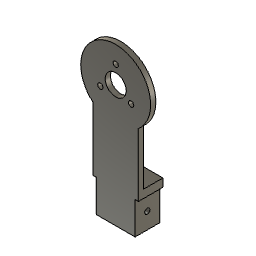
Upper structure (Autodesk Fusion 360 design; units mm, degrees)
Autodesk Fusion 360 part; units mm, degrees
sketch "Esquisse1" plane through (0, 0, 0) normal (0, 1, 0) x (1, 0, 0)
  circle A0 centre (0, -25) radius 21.6
  line L0 (0, 15.5) -> (14, 15.5)
  line L1 (0, 15.5) -> (-14, 15.5)
  line L2 (-14, 15.5) -> (-14, -8.5513)
  line L3 (14, 15.5) -> (14, -8.5513)
  circle A1 centre (0, -25) radius 6
  circle A2 centre (0, -36) radius 1.625
  circle A3 centre (-9.5263, -19.5) radius 1.625
  circle A4 centre (9.5263, -19.5) radius 1.625
  dimension "d1" = 43.2
  dimension "d4" = 14
  dimension "d5" = 14
  dimension "d9" = 11
  dimension "d12" = 12
  dimension "d64" = 3.25
  dimension "d65" = 3.25
  dimension "d66" = 3.25
  constraint coincident A0 L2.end
  constraint perpendicular L1 L2
  constraint coincident A0 L3.end
  constraint perpendicular L0 L3
  measures "d1" diameter of A0
  measures "d4" distance of L0.start L0.end
  measures "d5" distance of L0.start L1.end
  measures "d9" distance of A0.centre A4.centre
  measures "d12" diameter of A1
  measures "d64" diameter of A2
  measures "d65" diameter of A3
  measures "d66" diameter of A4
extrude "Extrusion1" add sketch "Esquisse1" along normal blind 3.2 contours A0 | A2 | A3 | A4
extrude "Extrusion2" add sketch "Esquisse1" along normal blind 3.2 contours A0 L0 L1 L2 L3
sketch "Esquisse2" plane through (0, 0, -15.5) normal (0, 0, -1) x (1, 0, 0)
  line L0 (14, 0) -> (-14, 0)
  line L1 (-14, 0) -> (-14, -3.2)
  line L2 (-14, -3.2) -> (14, -3.2)
  line L3 (14, -3.2) -> (14, 0)
  line L4 (-14, -3.2) -> (14, -3.2)
  dimension "d17" = 28
  constraint horizontal L4
  constraint coincident L1.end L2.start
  measures "d17" distance of L1.end L2.end
extrude "Extrusion3" add sketch "Esquisse2" along normal blind 10
sketch "Esquisse3" plane through (0, 0, -25.5) normal (0, 0, -1) x (1, 0, 0)
  line L0 (-14, 0) -> (-14, -3.2)
  line L1 (-14, -3.2) -> (14, -3.2)
  line L2 (14, -3.2) -> (14, 0)
  line L3 (14, 0) -> (-14, 0)
extrude "Extrusion4" cut sketch "Esquisse3" against normal blind 10
extrude "Extrusion5" add sketch "Esquisse2" along normal blind 5
sketch "Esquisse4" plane through (0, 0, -20.5) normal (0, 0, -1) x (1, 0, 0)
  line L0 (-14, -3.2) -> (14, -3.2)
  line L1 (14, -3.2) -> (14, 0)
  line L2 (14, 0) -> (-14, 0)
  line L3 (-14, 0) -> (-14, -3.2)
  line L4 (-14, -3.2) -> (-14, -15.2)
  line L5 (-14, -15.2) -> (14, -15.2)
  line L6 (14, -15.2) -> (14, -3.2)
  dimension "d25" = 12
  constraint vertical L4
  constraint horizontal L5
  constraint vertical L6
  constraint coincident L0.end L1.start
  measures "d25" distance of L0.end L5.end
extrude "Extrusion6" add sketch "Esquisse4" along normal blind 10
sketch "Esquisse5" plane through (0, 0, -20.5) normal (0, 0, 1) x (-1, 0, 0)
  line L0 (14, -3.2) -> (-14, -3.2)
  line L1 (-14, -3.2) -> (-14, -15.2)
  line L2 (-14, -15.2) -> (14, -15.2)
  line L3 (14, -15.2) -> (14, -3.2)
  line L4 (-14, -3.2) -> (-7.5, -3.2)
  line L5 (14, -3.2) -> (7.5, -3.2)
  line L6 (-7.5, -3.2) -> (-7.5, -6.7)
  line L7 (7.5, -3.2) -> (7.5, -6.7)
  circle A0 centre (-7.5, -6.7) radius 1.625
  circle A1 centre (7.5, -6.7) radius 1.625
  dimension "d28" = 6.5
  dimension "d29" = 6.5
  dimension "d32" = 3.5
  dimension "d33" = 3.5
  dimension "d34" = 3.25
  dimension "d35" = 3.25
  constraint coincident L0.end L1.start
  constraint perpendicular L1 L4
  constraint coincident L0.start L3.end
  constraint perpendicular L3 L5
  constraint perpendicular L0 L6
  constraint perpendicular L0 L7
  constraint coincident L6.end A0.centre
  constraint coincident L7.end A1.centre
  measures "d28" distance of L0.end L4.end
  measures "d29" distance of L0.start L5.end
  measures "d32" distance of L4.end L6.end
  measures "d33" distance of L5.end L7.end
  measures "d34" diameter of A0
  measures "d35" diameter of A1
extrude "Extrusion7" cut sketch "Esquisse5" against normal blind 8 contours A0
extrude "Extrusion8" cut sketch "Esquisse5" against normal blind 8 contours A1
sketch "Esquisse6" plane through (0, 0, -20.5) normal (0, 0, 1) x (-1, 0, 0)
  circle A0 centre (7.5, -6.7) radius 1.625
  circle A1 centre (-7.5, -6.7) radius 1.625
  line L0 (14, -3.2) -> (-14, -3.2)
  line L1 (-14, -3.2) -> (-14, -15.2)
  line L2 (-14, -15.2) -> (14, -15.2)
  line L3 (14, -15.2) -> (14, -3.2)
  line L4 (0, -3.2) -> (0, -10.7)
  dimension "d40" = 7.5
  constraint midpoint L0 L4.start
  constraint perpendicular L0 L4
  measures "d40" distance of L4.start L4.end
sketch "Esquisse7" plane through (0, 0, -30.5) normal (0, 0, -1) x (1, 0, 0)
  line L0 (14, -15.2) -> (14, 0)
  line L1 (14, 0) -> (-14, 0)
  line L2 (-14, 0) -> (-14, -15.2)
  line L3 (-14, -15.2) -> (14, -15.2)
  circle A0 centre (0, -7.6) radius 6.4
  circle A1 centre (0, -7.6) radius 3.865
  dimension "d56" = 7.73
  constraint concentric A0 A1
  measures "d56" diameter of A1
extrude "Extrusion9" add sketch "Esquisse7" along normal blind 20 contours A0 | A1
sketch "Esquisse8" plane through (0, 0, 0) normal (1, 0, 0) x (0, 1, 0)
sketch "Esquisse9" plane through (0, 0, 0) normal (0, 0, 1) x (1, 0, 0)
sketch "Esquisse10" plane through (0, 0, 0) normal (0, 0, 1) x (1, 0, 0)
sketch "Esquisse11" plane through (0, 0, 0) normal (1, 0, 0) x (0, 1, 0)
sketch "Esquisse12" plane through (-14, 0, 0) normal (-1, 0, 0) x (0, -1, 0)
  line L0 (0, -30.5) -> (0, 8.5513)
  line L1 (0, 8.5513) -> (-3.2, 8.5513)
  line L2 (-3.2, 8.5513) -> (-3.2, -20.5)
  line L3 (-3.2, -20.5) -> (-15.2, -20.5)
  line L4 (-15.2, -20.5) -> (-15.2, -30.5)
  line L5 (-15.2, -30.5) -> (0, -30.5)
  line L6 (-15.2, -25.5) -> (-7.6, -25.5)
  line L7 (-7.6, -25.5) -> (-7.6, -40.5)
  circle A0 centre (-7.6, -40.5) radius 1.625
  dimension "d44" = 7.6
  dimension "d45" = 15
  dimension "d46" = 3.25
  constraint midpoint L4 L6.start
  constraint perpendicular L4 L6
  constraint perpendicular L5 L7
  constraint coincident L7.end A0.centre
  measures "d44" distance of L6.start L6.end
  measures "d45" distance of L6.end L7.end
  measures "d46" diameter of A0
extrude "Extrusion10" cut sketch "Esquisse12" against normal blind 30 contours A0
sketch "Esquisse13" plane through (0, 0, 0) normal (0, 0, 1) x (1, 0, 0)
sketch "Esquisse14" plane through (0, 3.2, 0) normal (0, 1, 0) x (-1, 0, 0)
  line L0 (14, -20.5) -> (14, 8.5513)
  arc A0 (14, 8.5513) -> (-14, 8.5513) centre (0, 25) ccw
  line L1 (-14, 8.5513) -> (-14, -20.5)
  line L2 (-14, -20.5) -> (14, -20.5)
  circle A1 centre (0, 25) radius 6
  circle A2 centre (0, 25) radius 6
  constraint concentric A0 A2
extrude "Extrusion11" add sketch "Esquisse14" against normal blind 3.2 contours A1 A2
sketch "Esquisse15" plane through (0, 3.2, 0) normal (0, 1, 0) x (-1, 0, 0)
  line L0 (14, -20.5) -> (14, 8.5513)
  arc A0 (14, 8.5513) -> (-14, 8.5513) centre (0, 25) ccw
  line L1 (-14, 8.5513) -> (-14, -20.5)
  line L2 (-14, -20.5) -> (14, -20.5)
  circle A1 centre (0, 25) radius 6.5
  dimension "d51" = 13
  constraint concentric A0 A1
  measures "d51" diameter of A1
extrude "Extrusion12" cut sketch "Esquisse15" against normal blind 3.2 contours A1
extrude "Extrusion13" cut 1 faces at (-1.5877, 5.831, -50.5) along direction (0, 0, 1) blind 20
extrude "Extrusion14" add sketch "Esquisse7" along normal blind 20 contours A0
sketch "Esquisse16" plane through (-14, 0, 0) normal (-1, 0, 0) x (0, -1, 0)
  line L0 (0, -30.5) -> (0, 8.5513)
  line L1 (0, 8.5513) -> (-3.2, 8.5513)
  line L2 (-3.2, 8.5513) -> (-3.2, -20.5)
  line L3 (-3.2, -20.5) -> (-15.2, -20.5)
  line L4 (-15.2, -20.5) -> (-15.2, -30.5)
  line L5 (-15.2, -30.5) -> (0, -30.5)
  line L6 (-15.2, -25.5) -> (-15, -25.5)
  circle A0 centre (-7.7, -40.5) radius 1.625
  dimension "d61" = 3.25
  constraint midpoint L4 L6.start
  constraint perpendicular L4 L6
  measures "d61" diameter of A0
extrude "Extrusion15" cut sketch "Esquisse16" against normal blind 30 contours A0
extrude "Extrusion16" cut sketch "Esquisse1" along normal blind 3.2 contours A2
extrude "Extrusion17" cut sketch "Esquisse1" along normal blind 3.2 contours A3
extrude "Extrusion18" cut sketch "Esquisse1" along normal blind 3.2 contours A4
extrude "Extrusion19" cut 1 faces at (5.5168, 8.11, -50.5) along direction (0, 0, 1) blind 20
sketch "Esquisse17" plane through (0, 0, -30.5) normal (0, 0, -1) x (1, 0, 0)
  line L0 (14, -15.2) -> (14, 0)
  line L1 (14, 0) -> (-14, 0)
  line L2 (-14, 0) -> (-14, -15.2)
  line L3 (-14, -15.2) -> (14, -15.2)
  circle A0 centre (0, -7.6) radius 3.865
  line L4 (-12, 0) -> (12, 0)
  line L5 (12, 0) -> (12, -15.2)
  line L6 (12, -15.2) -> (-12, -15.2)
  line L7 (-12, -15.2) -> (-12, 0)
  dimension "d75" = 7.73
  dimension "d76" = 24
  constraint horizontal L4
  constraint vertical L5
  constraint horizontal L6
  constraint vertical L7
  constraint coincident L1 L4.start
  measures "d75" diameter of A0
  measures "d76" distance of L4.start L4.end
sketch "Esquisse18" plane through (14, 0, 0) normal (1, 0, 0) x (0, 1, 0)
  line L0 (3.2, -20.5) -> (3.2, 8.5513)
  line L1 (3.2, 8.5513) -> (0, 8.5513)
  line L2 (0, 8.5513) -> (0, -30.5)
  line L3 (0, -30.5) -> (15.2, -30.5)
  line L4 (15.2, -30.5) -> (15.2, -20.5)
  line L5 (15.2, -20.5) -> (3.2, -20.5)
extrude "Extrusion20" add sketch "Esquisse17" along normal blind 20 contours L1 L3 L4 L5 L6 L7
sketch "Esquisse19" plane through (12, 0, 0) normal (1, 0, 0) x (0, 1, 0)
  line L0 (15.2, -30.5) -> (0, -30.5)
  line L1 (0, -30.5) -> (0, -50.5)
  line L2 (0, -50.5) -> (15.2, -50.5)
  line L3 (15.2, -50.5) -> (15.2, -30.5)
extrude "Extrusion21" cut 1 faces at (-2.3021, 12.8709, -20.5) along direction (0, 0, -1) blind 5
extrude "Extrusion22" cut 1 faces at (-8.0356, 6.7807, -28.5) along direction (0, 0, -1) blind 2
extrude "Extrusion23" cut 1 faces at (6.9644, 7.5176, -28.5) along direction (0, 0, -1) blind 2
sketch "Esquisse20" plane through (12, 0, 0) normal (1, 0, 0) x (0, 1, 0)
sketch "Esquisse21" plane through (12, 0, 0) normal (1, 0, 0) x (0, 1, 0)
sketch "Esquisse22" plane through (-12, 0, 0) normal (-1, 0, 0) x (0, -1, 0)
  line L0 (0, -30.5) -> (-15.2, -30.5)
  line L1 (-15.2, -30.5) -> (-15.2, -50.5)
  line L2 (-15.2, -50.5) -> (0, -50.5)
  line L3 (0, -50.5) -> (0, -30.5)
  line L4 (-15.2, -40.5) -> (0, -40.5)
  line L5 (-7.6, -50.5) -> (-7.6, -30.5)
  constraint midpoint L1 L4.start
  constraint midpoint L3 L4.end
  constraint midpoint L2 L5.start
  constraint midpoint L0 L5.end
hole "Perçage2" at (-12, 7.5778, -40.5226) direction (1, 0, 0) diameter 3.25 depth 30 tip angle 118
sketch "Esquisse23" plane through (0, 0, -50.5) normal (0, 0, -1) x (1, 0, 0)
  circle A0 centre (0, -7.6) radius 3.865
  line L0 (-12, -15.2) -> (12, -15.2)
  line L1 (12, -15.2) -> (12, 0)
  line L2 (12, 0) -> (-12, 0)
  line L3 (-12, 0) -> (-12, -15.2)
  line L4 (-12, -7.6) -> (12, -7.6)
  line L5 (-12, -7.6) -> (-7.9325, -7.6)
  line L6 (12, -7.6) -> (7.9325, -7.6)
  line L7 (-7.9325, -7.6) -> (-6.5325, -7.6)
  line L8 (-7.9325, -7.6) -> (-9.3325, -7.6)
  line L9 (-9.3325, -7.6) -> (-9.3325, -4.7)
  line L10 (-9.3325, -7.6) -> (-9.3325, -10.5)
  line L11 (-9.3325, -4.7) -> (-6.5325, -4.7)
  line L12 (-6.5325, -4.7) -> (-6.5325, -10.5)
  line L13 (-6.5325, -10.5) -> (-9.3325, -10.5)
  line L14 (-9.3325, -10.5) -> (-9.3325, -4.7)
  line L15 (7.9325, -7.6) -> (6.5325, -7.6)
  line L16 (6.5325, -7.6) -> (6.5325, -4.7)
  line L17 (6.5325, -4.7) -> (9.3325, -4.7)
  line L18 (9.3325, -4.7) -> (9.3325, -10.5)
  line L19 (9.3325, -10.5) -> (6.5325, -10.5)
  line L20 (6.5325, -10.5) -> (6.5325, -4.7)
  dimension "d92" = 4.0675
  dimension "d94" = 1.4
  dimension "d95" = 2.9
  dimension "d96" = 2.9
  dimension "d97" = 2.8
  dimension "d98" = 5.8
  dimension "d99" = 1.4
  dimension "d100" = 2.9
  dimension "d101" = 2.8
  dimension "d102" = 5.8
  constraint midpoint L3 L4.start
  constraint midpoint L1 L4.end
  constraint perpendicular L3 L5
  constraint perpendicular L1 L6
  constraint parallel L4 L7
  constraint parallel L5 L8
  constraint perpendicular L4 L9
  constraint perpendicular L5 L10
  constraint horizontal L11
  constraint vertical L12
  constraint horizontal L13
  constraint vertical L14
  constraint parallel L4 L15
  constraint perpendicular L15 L16
  constraint horizontal L17
  constraint vertical L18
  constraint horizontal L19
  constraint vertical L20
  measures "d92" distance of L4.end L6.end
  measures "d94" distance of L5.end L8.end
  measures "d95" distance of L8.end L9.end
  measures "d96" distance of L8.end L10.end
  measures "d97" distance of L9.end L11.end
  measures "d98" distance of L9.end L10.end
  measures "d99" distance of L6.end L15.end
  measures "d100" distance of L15.end L16.end
  measures "d101" distance of L16.end L17.end
  measures "d102" distance of L16.end L19.end
ref_plane "Plan de construction1" through (-7.9325, 7.6, -50.5) normal (1, 0, 0) x (0, 1, 0)
sketch "Esquisse24" plane through (-7.9325, 7.6, -50.5) normal (1, 0, 0) x (0, 1, 0)
  line L0 (0, 6.8) -> (2.7713, 8.4)
  line L1 (2.7713, 8.4) -> (2.7713, 11.6)
  line L2 (2.7713, 11.6) -> (0, 13.2)
  line L3 (0, 13.2) -> (-2.7713, 11.6)
  line L4 (-2.7713, 11.6) -> (-2.7713, 8.4)
  line L5 (-2.7713, 8.4) -> (0, 6.8)
  point P0 (0, 10)
  dimension "d104" = 3.2
  measures "d104" distance of L0.start P0
extrude "Extrusion24" cut sketch "Esquisse24" against normal blind 1.4
extrude "Extrusion25" cut sketch "Esquisse24" along normal blind 1.4
extrude "Extrusion26" cut sketch "Esquisse23" against normal blind 10 contours L4 L5 L7 L8 L10 L12 L13 L14 | L4 L5 L7 L8 L9 L11 L12 L14
ref_plane "Plan de construction2" through (7.9325, 7.6, -50.5) normal (1, 0, 0) x (0, 1, 0)
sketch "Esquisse25" plane through (7.9325, 7.6, -50.5) normal (1, 0, 0) x (0, 1, 0)
  line L0 (0, 6.8) -> (2.7713, 8.4)
  line L1 (2.7713, 8.4) -> (2.7713, 11.6)
  line L2 (2.7713, 11.6) -> (0, 13.2)
  line L3 (0, 13.2) -> (-2.7713, 11.6)
  line L4 (-2.7713, 11.6) -> (-2.7713, 8.4)
  line L5 (-2.7713, 8.4) -> (0, 6.8)
  point P0 (0, 10)
  dimension "d112" = 3.2
  measures "d112" distance of L0.start P0
extrude "Extrusion27" cut sketch "Esquisse25" along normal blind -1.2 and the other way blind -1.2
extrude "Extrusion28" cut sketch "Esquisse23" against normal blind 10 contours L4 L6 L15 L16 L17 L18 L20 | L4 L6 L15 L18 L19 L20
extrude "Extrusion29" cut 1 faces at (6.9644, 7.5176, -30.5) along direction (0, 0, -1) blind 4
extrude "Extrusion30" cut 1 faces at (-8.0356, 6.7807, -30.5) along direction (0, 0, -1) blind 4
sketch "Esquisse26" plane through (0, 0, -25.5) normal (0, 0, 1) x (-1, 0, 0)
  circle A0 centre (7.5, -6.7) radius 1.625
  circle A1 centre (-7.5, -6.7) radius 1.625
  line L0 (14, -3.2) -> (-14, -3.2)
  line L1 (-14, -3.2) -> (-14, -15.2)
  line L2 (-14, -15.2) -> (14, -15.2)
  line L3 (14, -15.2) -> (14, -3.2)
  line L4 (-7.5, -6.7) -> (-7.5, -15.2)
  line L5 (7.5, -6.7) -> (7.5, -15.2)
  constraint coincident A1.centre L4.start
  constraint coincident L2 L4.end
  constraint perpendicular L2 L4
  constraint coincident A0.centre L5.start
  constraint coincident L2 L5.end
  constraint perpendicular L2 L5
sketch "Esquisse27" plane through (0, 15.2, 0) normal (0, 1, 0) x (-1, 0, 0)
  line L0 (14, -25.5) -> (-14, -25.5)
  line L1 (-14, -25.5) -> (-14, -30.5)
  line L2 (-14, -30.5) -> (-12, -30.5)
  line L3 (-12, -30.5) -> (-12, -50.5)
  line L4 (-12, -50.5) -> (12, -50.5)
  line L5 (12, -50.5) -> (12, -30.5)
  line L6 (12, -30.5) -> (14, -30.5)
  line L7 (14, -30.5) -> (14, -25.5)
  line L8 (-12, -31) -> (-7.5, -31)
  line L9 (12, -31) -> (7.5, -31)
  dimension "d123" = 4.5
  dimension "d124" = 4.5
  constraint coincident L3 L8.start
  constraint perpendicular L3 L8
  constraint coincident L5 L9.start
  constraint perpendicular L5 L9
  measures "d123" distance of L8.start L8.end
  measures "d124" distance of L9.start L9.end
sketch "Esquisse28" plane through (0, 0, -25.5) normal (0, 0, 1) x (-1, 0, 0)
  circle A0 centre (7.5, -6.7) radius 1.625
  circle A1 centre (-7.5, -6.7) radius 1.625
  line L0 (14, -3.2) -> (-14, -3.2)
  line L1 (-14, -3.2) -> (-14, -15.2)
  line L2 (-14, -15.2) -> (14, -15.2)
  line L3 (14, -15.2) -> (14, -3.2)
  line L4 (7.5, -6.7) -> (7.5, -15.2)
  constraint coincident A0.centre L4.start
  constraint coincident L2 L4.end
  constraint perpendicular L2 L4
ref_plane "Plan de construction3" through (0, 9.2, -30.5) normal (0, 0, 1) x (-1, 0, 0)
sketch "Esquisse29" plane through (0, 0, -30.5) normal (0, 0, 1) x (1, 0, 0)
  line L0 (5.8679, 3.9475, 5) -> (9.0677, 3.9103, 5)
  line L1 (9.0677, 3.9103, 5) -> (10.6998, 6.6628, 5)
  line L2 (10.6998, 6.6628, 5) -> (9.1321, 9.4525, 5)
  line L3 (9.1321, 9.4525, 5) -> (5.9323, 9.4897, 5)
  line L4 (5.9323, 9.4897, 5) -> (4.3002, 6.7372, 5)
  line L5 (4.3002, 6.7372, 5) -> (5.8679, 3.9475, 5)
  line L6 (-9.1264, 3.9441) -> (-5.9265, 3.9136)
  line L7 (-5.9265, 3.9136) -> (-4.3001, 6.6695)
  line L8 (-4.3001, 6.6695) -> (-5.8736, 9.4559)
  line L9 (-5.8736, 9.4559) -> (-9.0735, 9.4864)
  line L10 (-9.0735, 9.4864) -> (-10.6999, 6.7305)
  line L11 (-10.6999, 6.7305) -> (-9.1264, 3.9441)
  point P0 (7.5, 6.7)
  point P1 (-7.5, 6.7)
  dimension "d126" = 3.2
  dimension "d127" = 3.2
  measures "d127" distance of L6.start P1
sketch "Esquisse30" plane through (0, 0, -30.5) normal (0, 0, 1) x (1, 0, 0)
  line L0 (5.9553, 9.5025) -> (4.3006, 6.7635)
  line L1 (4.3006, 6.7635) -> (5.8453, 3.961)
  line L2 (5.8453, 3.961) -> (9.0447, 3.8975)
  line L3 (9.0447, 3.8975) -> (10.6994, 6.6365)
  line L4 (10.6994, 6.6365) -> (9.1547, 9.439)
  line L5 (9.1547, 9.439) -> (5.9553, 9.5025)
  line L6 (-5.8991, 9.4707) -> (-9.0991, 9.4718)
  line L7 (-9.0991, 9.4718) -> (-10.7, 6.7011)
  line L8 (-10.7, 6.7011) -> (-9.1009, 3.9293)
  line L9 (-9.1009, 3.9293) -> (-5.9009, 3.9282)
  line L10 (-5.9009, 3.9282) -> (-4.3, 6.6989)
  line L11 (-4.3, 6.6989) -> (-5.8991, 9.4707)
  point P0 (7.5, 6.7)
  point P1 (-7.5, 6.7)
  dimension "d128" = 3.2
  dimension "d129" = 3.2
  measures "d128" distance of L0.start P0
  measures "d129" distance of L6.start P1
extrude "Extrusion31" cut sketch "Esquisse30" along normal blind 1.4 and the other way blind 1.4 contours L0 L1 L2 L3 L4 L5
extrude "Extrusion32" cut sketch "Esquisse30" along normal blind 1.4 and the other way blind 1.4 contours L6 L7 L8 L9 L10 L11
sketch "Esquisse31" plane through (0, 15.2, 0) normal (0, 1, 0) x (-1, 0, 0)
  line L0 (14, -25.5) -> (-14, -25.5)
  line L1 (-14, -25.5) -> (-14, -30.5)
  line L2 (-14, -30.5) -> (-12, -30.5)
  line L3 (-12, -30.5) -> (-12, -50.5)
  line L4 (-12, -50.5) -> (12, -50.5)
  line L5 (12, -50.5) -> (12, -30.5)
  line L6 (12, -30.5) -> (14, -30.5)
  line L7 (14, -30.5) -> (14, -25.5)
  line L8 (-4.6, -30.5) -> (-4.6, -29.1)
  line L9 (10.4, -29.1) -> (4.6, -29.1)
  line L10 (-4.6, -29.1) -> (-10.4, -29.1)
  line L11 (-10.4, -29.1) -> (-10.4, -31.9)
  line L12 (-10.4, -31.9) -> (-4.6, -31.9)
  line L13 (-4.6, -31.9) -> (-4.6, -29.1)
  line L14 (4.6, -29.1) -> (4.6, -31.9)
  line L15 (4.6, -31.9) -> (10.4, -31.9)
  line L16 (10.4, -31.9) -> (10.4, -29.1)
  dimension "d139" = 1.4
  dimension "d143" = 5.8
  dimension "d145" = 5.8
  dimension "d146" = 2.8
  dimension "d147" = 2.8
  constraint horizontal L9
  constraint horizontal L10
  constraint vertical L11
  constraint horizontal L12
  constraint vertical L13
  constraint vertical L14
  constraint horizontal L15
  constraint vertical L16
  measures "d139" distance of L8.start L8.end
  measures "d143" distance of L9.start L9.end
  measures "d145" distance of L8.end L10.end
  measures "d146" distance of L8.end L12.end
  measures "d147" distance of L9.start L15.end
extrude "Extrusion33" cut sketch "Esquisse31" against normal blind 9 contours L8 L10 L11 L12 L13
extrude "Extrusion34" cut sketch "Esquisse31" against normal blind 9 contours L9 L14 L15 L16
